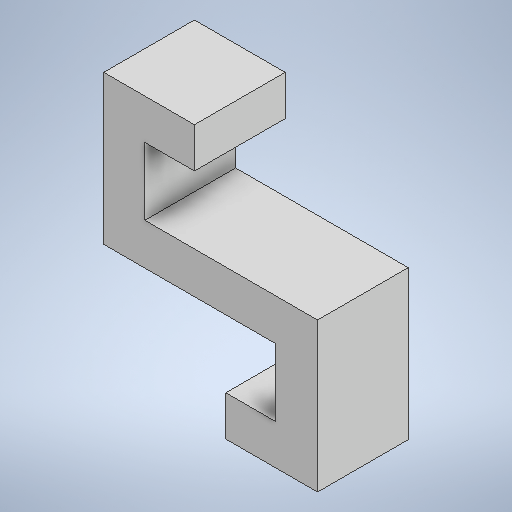
# Autodesk Inventor part: Haken für Bioprinter 4x9mm 001
Saved by Autodesk Inventor 2025 (Build 290162000, 162)
## iProperties
Created: 2024-04-08
Part Number: Haken für Bioprinter 4x9mm 001
Material: Generisch
Document SubType Name: Modeling
Designer: noahm
Density: 1 g/cm^3
Appearance: Vorgabe
Author: noahm
Autodesk Inventor part; units mm, degrees
ref_plane "YZ Plane" through (0, 0, 0) normal (1, 0, 0) x (0, 1, 0)
ref_plane "XZ Plane" through (0, 0, 0) normal (0, 1, 0) x (-1, 0, 0)
ref_plane "XY Plane" through (0, 0, 0) normal (0, 0, 1) x (1, 0, 0)
sketch "Skizze1" plane through (0, 0, 0) normal (0, 1, 0) x (-1, 0, 0)
  line L0 (-10.1354, -12.1625) -> (-1.4354, -12.1625)
  line L1 (10.1354, -1.9625) -> (10.1354, 12.1625)
  line L2 (10.1354, 12.1625) -> (1.5354, 12.1625)
  line L3 (-10.1354, 1.9625) -> (-10.1354, -12.1625)
  line L4 (-10.1354, -12.1625) -> (10.1354, 12.1625) construction
  line L5 (10, -12) -> (-10, 12) construction
  line L6 (1.5354, 12.1625) -> (1.5354, 8.3625)
  line L7 (1.5354, 8.3625) -> (6.2354, 8.3625)
  line L8 (6.2354, 8.3625) -> (6.2354, 1.9625)
  line L9 (6.2354, 1.9625) -> (-10.1354, 1.9625)
  line L10 (-1.4354, -12.1625) -> (-1.4354, -8.3625)
  line L11 (-1.4354, -8.3625) -> (-6.1354, -8.3625)
  line L12 (-6.1354, -8.3625) -> (-6.1354, -1.9625)
  line L13 (-6.1354, -1.9625) -> (10.1354, -1.9625)
  point P0 (0, 0)
  point P1 (1.5354, 10.2625)
  point P2 (6.2354, 5.1625)
  point P3 (-1.4354, -10.2625)
  dimension "d12" = 6.4
  dimension "d13" = 3.8
  dimension "d14" = 6.4
  dimension "d15" = 3.925
  dimension "d16" = 3.9
  dimension "d17" = 3.8
  dimension "d18" = 4.7
  dimension "d19" = 4.7
  constraints: 28 end point, 5 midpoint, 5 perpendicular, 4 parallel, 3 horizontal
  measures "d12" distance between parallel lines of L9 L7
  measures "d13" distance between parallel lines of L0 L11
  measures "d14" distance between parallel lines of L13 L11
  measures "d15" distance between parallel lines of L13 L9
  measures "d16" distance between parallel lines of L1 L8
  measures "d17" distance between parallel lines of L2 L7
  measures "d18" distance of L10.end L11.end
  measures "d19" distance of L6.end L7.end
extrude "Extrusion1" add sketch "Skizze1" along normal blind 8.6
